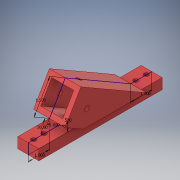
# Autodesk Inventor part: 30degreeAttachement
Saved by Autodesk Inventor 2019.3 (Build 233278000, 278)
## iProperties
Created: 2019-02-15
Part Number: 30degreeAttachement
Material: PBT Plastic
Document SubType Name: Modeling
Designer: steele
Density: 1.31 g/cm^3
Appearance: Smooth - Red
Author: steele
Autodesk Inventor part; units mm, degrees
note: some values were not read from the file. Chosen so that the rebuilt part matches the saved one: direction of "Hole2".
ref_plane "YZ Plane" through (0, 0, 0) normal (1, 0, 0) x (0, 1, 0)
ref_plane "XZ Plane" through (0, 0, 0) normal (0, 1, 0) x (-1, 0, 0)
ref_plane "XY Plane" through (0, 0, 0) normal (0, 0, 1) x (1, 0, 0)
sketch "Sketch1" plane through (0, 0, 0) normal (1, 0, 0) x (0, 1, 0)
  line L0 (0, 0) -> (12.7, 21.997)
  line L1 (0, 0) -> (0, 47.397)
  line L2 (0, 0) -> (0, -101.6)
  line L3 (12.7, 21.997) -> (45.6956, 2.947)
  line L4 (45.6956, 2.947) -> (0, -76.2)
  line L5 (12.7, 21.997) -> (0, 21.997) construction
  line L6 (0, 47.397) -> (-12.7, 47.397)
  line L7 (-12.7, 47.397) -> (-12.7, -76.2)
  line L8 (0, -101.6) -> (-12.7, -101.6)
  line L9 (-12.7, -101.6) -> (-12.7, -76.2)
  dimension "d0" = 38.1
  dimension "d1" = 25.4
  dimension "d6" = 30
  dimension "d7" = 25.4
  dimension "d21" = 25.4
  dimension "d22" = 12.7
  constraints: 20 end point, 4 perpendicular, 2 horizontal, 2 point on line, 2 vertical, 1 parallel
  measures "d0" distance of L0.end L3.end
  measures "d1" distance of L0.end L0.start
  measures "d6" angle of L0 L1
  measures "d7" distance from line of L1.end L5
  measures "d21" distance from line of L8 L4.end
  measures "d22" distance between parallel lines of L7 L2
extrude "Extrusion2" add sketch "Sketch1" along normal mid plane 38.1 contours L0 L3 L4 L2
extrude "Extrusion3" add sketch "Sketch1" along normal mid plane 25.4
sketch "Sketch2" plane through (-19.05, 12.7, 21.997) normal (0, 0.5, 0.8660254) x (1, 0, 0)
  line L0 (32.385, 5.715) -> (32.385, 32.385)
  line L1 (32.385, 32.385) -> (5.715, 32.385)
  line L2 (5.715, 32.385) -> (5.715, 5.715)
  line L3 (5.715, 5.715) -> (32.385, 5.715)
  line L4 (32.385, 5.715) -> (5.715, 32.385) construction
  line L5 (32.385, 32.385) -> (5.715, 5.715) construction
  line L6 (0, 0) -> (0, 38.1) projected
  line L7 (38.1, 38.1) -> (38.1, 0) projected
  line L8 (0, 38.1) -> (38.1, 38.1) projected
  point P0 (19.05, 0)
  point P1 (19.05, 19.05)
  dimension "d16" = 26.67
  dimension "d17" = 19.05
  dimension "d18" = 19.05
  constraints: 12 end point, 3 parallel, 2 midpoint, 2 perpendicular
  measures "d16" distance of L0.end L1.end
  measures "d17" distance from line of point (19.05, 19.05) L7
  measures "d18" distance from line of point (19.05, 19.05) L8
extrude "Extrusion4" cut sketch "Sketch2" against normal blind 38.1
sketch "Sketch3" plane through (-12.7, 0, 47.397) normal (0, 1, 0) x (1, 0, 0)
  point P0 (12.7, 47.397)
sketch "Sketch4" plane through (-12.7, 0, 47.397) normal (0, 1, 0) x (1, 0, 0)
  line L0 (25.4, 0) -> (0, 0) projected
  line L1 (-6.35, 25.4) -> (31.75, 25.4) projected
  line L2 (0, 123.597) -> (25.4, 123.597) projected
  line L3 (25.4, 148.997) -> (0, 148.997) projected
  point P0 (12.7, 47.397)
  point P1 (12.7, 6.35)
  point P2 (12.7, 19.05)
  point P3 (12.7, 129.947)
  point P4 (12.7, 142.647)
  dimension "d23" = 6.35
  dimension "d24" = 6.35
  dimension "d25" = 6.35
  dimension "d26" = 6.35
  measures "d23" distance from line of point (12.7, 6.35) L0
  measures "d24" distance from line of point (12.7, 19.05) L1
  measures "d25" distance from line of point (12.7, 129.947) L2
  measures "d26" distance from line of L3 point (12.7, 142.647)
hole "Hole1" at (0, 0, 41.047) at (0, 0, 28.347) at (0, 0, -82.55) at (0, 0, -95.25) direction (0, -1, 0) diameter 5.6134 end through all clearance for "Flat Head Machine Screw (82)" size "#10" standard "Ansi Unified Screw Threads"
sketch "Sketch5" plane through (19.05, 0, 0) normal (1, 0, 0) x (0, 0, -1)
  line L0 (-21.997, 12.7) -> (-2.947, 45.6956) construction
  line L1 (-12.472, 29.1978) -> (38.1, 0) construction
  line L2 (0, 0) -> (76.2, 0) construction
  line L3 (-21.997, 12.7) -> (0, 0) construction
  point P0 (4.0257, 19.6728)
  dimension "d34" = 19.05
  constraints: 2 end point, 2 midpoint, 1 parallel, 1 point on line
  measures "d34" distance from line of L0 point (4.026, 19.673)
sketch "Sketch6" plane through (-19.05, 45.6956, 2.947) normal (0, 0.8660254, -0.5) x (1, 0, 0)
  line L0 (0, 0) -> (38.1, 0) projected
  point P0 (19.05, 25.4)
  point P1 (19.05, 19.05)
  dimension "d35" = 19.05
  measures "d35" distance from line of point (19.05, 19.05) L0
hole "Hole2" at (0, 36.1706, -13.5507) direction (0, -0.8660254, 0.5) diameter 5.6134 depth 5.715 clearance for "Flat Head Machine Screw (82)" size "#10" standard "Ansi Unified Screw Threads"
hole "Hole3" at (19.05, 19.6728, -4.0257) direction (-1, 0, 0) diameter 5.6134 end through all clearance for "Flat Head Machine Screw (82)" size "#10" standard "Ansi Unified Screw Threads"
body "Solid2"
